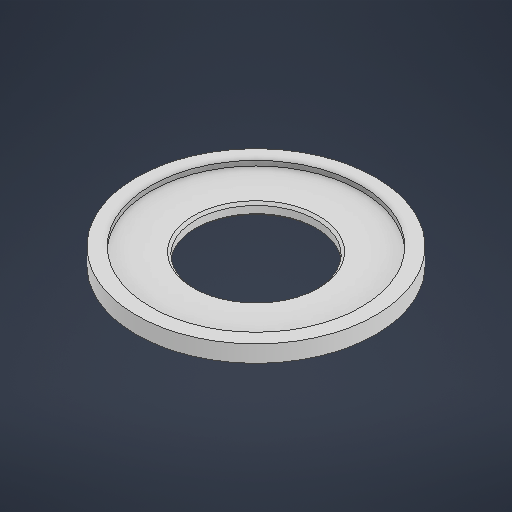
# Autodesk Inventor part: clutch for print
Saved by Autodesk Inventor 2025.2 (Build 292293000, 293)
## iProperties
Created: 2025-04-19
Part Number: clutch for print
Material: Generic
Document SubType Name: Modeling
Designer: klawy
Density: 1 g/cm^3
Appearance: Default
Author: klawy
Autodesk Inventor part; units mm, degrees
ref_plane "YZ Plane" through (0, 0, 0) normal (1, 0, 0) x (0, 1, 0)
ref_plane "XZ Plane" through (0, 0, 0) normal (0, 1, 0) x (-1, 0, 0)
ref_plane "XY Plane" through (0, 0, 0) normal (0, 0, 1) x (1, 0, 0)
sketch "Sketch2" plane through (0, 0, 0) normal (0, 0, 1) x (1, 0, 0)
  line L0 (12.6, 0) -> (25, 0)
  line L1 (25, 0) -> (25, 2.5)
  line L2 (25, 2.5) -> (12.6, 2.5)
  line L3 (12.6, 2.5) -> (12.6, 0)
  line L4 (25, 2.5) -> (22, 2.5)
  line L5 (22, 2.5) -> (22, 3.5)
  line L6 (22, 3.5) -> (25, 3.5)
  line L7 (25, 3.5) -> (25, 2.5)
  line L8 (0, -9.1355) -> (0, 9.1355) construction
  line L9 (25, 2.5) -> (22.5, 2.5)
  line L10 (22.5, 0) -> (25, 0)
  line L11 (25, 0) -> (25, 2.5)
  point P0 (0, 0)
  dimension "d4" = 12.6
  dimension "d6" = 2.5
  dimension "d7" = 3
  dimension "d8" = 1
  dimension "d15" = 25
  constraints: 24 end point, 5 parallel, 3 horizontal, 2 perpendicular, 2 point on line, 1 midpoint, 1 vertical
  measures "d4" distance from line of point (0, 0) L3
  measures "d6" distance from line of L0.end L2
  measures "d7" distance of L5.end L6.end
  measures "d8" distance between parallel lines of L6 L2
  measures "d15" distance from line of point (0, 0) L7
revolve "Revolution1" add sketch "Sketch2" angle 360 about axis through (0, -9.1355, 0) along (0, 1, 0)
chamfer "Chamfer1" distance 0.5 angle 45 2 edges at (-12.6, 2.5, 0) (-12.6, 0, 0)
body "Solid1"
